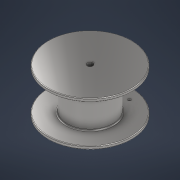
# Autodesk Inventor part: reel
Saved by Autodesk Inventor 2021 (Build 250183000, 183)
## iProperties
Created: 2021-06-19
Part Number: reel
Material: Stainless Steel
Document SubType Name: Modeling
Designer: Watchdog
Density: 8 g/cm^3
Appearance: Semi-Polished
Author: Watchdog
Autodesk Inventor part; units mm, degrees
ref_plane "YZ Plane" through (0, 0, 0) normal (1, 0, 0) x (0, 1, 0)
ref_plane "XZ Plane" through (0, 0, 0) normal (0, 1, 0) x (-1, 0, 0)
ref_plane "XY Plane" through (0, 0, 0) normal (0, 0, 1) x (1, 0, 0)
sketch "Sketch1" plane through (0, 0, 0) normal (0, 0, 1) x (1, 0, 0)
  line L0 (0, 70) -> (-66, 70)
  line L1 (-66, 70) -> (-66, 65)
  line L2 (-66, 65) -> (-36, 65)
  line L3 (-36, 65) -> (-36, 5)
  line L4 (-36, 5) -> (-66, 5)
  line L5 (-66, 5) -> (-66, 0)
  line L6 (-66, 0) -> (0, 0)
  line L7 (0, 0) -> (0, 70)
  dimension "d0" = 5
  dimension "d1" = 5
  dimension "d2" = 66
  dimension "d3" = 36
  dimension "d4" = 60
  constraints: 16 end point, 6 perpendicular, 2 point on line, 1 horizontal
  measures "d0" distance between parallel lines of L2 L0
  measures "d1" distance between parallel lines of L6 L4
  measures "d2" distance between parallel lines of L7 L1
  measures "d3" distance between parallel lines of L7 L3
  measures "d4" distance between parallel lines of L4 L2
revolve "Revolution1" add sketch "Sketch1" angle 360 about axis through (0, 0, 0) along (0, 1, 0)
fillet "Fillet1" radius 2 2 edges at (36, 5, 0) (36, 65, 0)
fillet "Fillet2" radius 1 4 edges at (66, 70, 0) (66, 65, 0) (66, 5, 0) (66, 0, 0)
sketch "Sketch2" plane through (0, 70, 0) normal (0, 1, 0) x (1, 0, 0)
  circle A0 centre (0, 0) radius 4.5
  line L0 (-1.5, 4.2426) -> (1.5, 4.2426)
  line L1 (1.5, 4.2426) -> (1.5, 5.8)
  line L2 (1.5, 5.8) -> (-1.5, 5.8)
  line L3 (-1.5, 5.8) -> (-1.5, 4.2426)
  dimension "d8" = 9
  dimension "d9" = 5.8
  dimension "d10" = 3
  constraints: 8 end point, 2 parallel, 2 point on circle, 1 centre point, 1 coincident, 1 horizontal, 1 perpendicular
  measures "d8" diameter of A0
  measures "d9" distance from line of point (0, 0) L2
  measures "d10" distance between parallel lines of L3 L1
extrude "Extrusion1" cut sketch "Sketch2" against normal blind 18
sketch "Sketch3" plane through (0, 0, 0) normal (0, -1, 0) x (1, 0, 0)
  point P0 (0, 0)
  point P1 (14.4669, -47.8614)
  point P2 (-34.2157, -36.4594)
  dimension "d13" = 50
  dimension "d14" = 50
  dimension "d15" = 50
  measures "d13" distance of point (0, 0) point (14.467, -47.861)
  measures "d14" distance of point (0, 0) point (-34.216, -36.459)
  measures "d15" distance of point (-34.216, -36.459) point (14.467, -47.861)
hole "Hole1" at (14.4669, 0, -47.8614) at (-34.2157, 0, -36.4594) direction (0, 1, 0) diameter 5 depth 8
ref_plane "midPlane" through (0, 35, 0) normal (0, 1, 0) x (1, 0, 0)
sketch "Sketch4" plane through (0, 0, 0) normal (0, -1, 0) x (1, 0, 0)
  circle A0 centre (0, 0) radius 11
  point P0 (0, 0)
  dimension "d23" = 22
  constraints: 1 centre point, 1 coincident
  measures "d23" diameter of A0
extrude "Extrusion2" cut sketch "Sketch4" against normal blind 7.5
chamfer "Chamfer1" distance 0.5 angle 45 1 edges at (-11, 0, 0)
equation "\"d1\" = d0"
equation "\"d14\" = d13"
body "Solid1"
